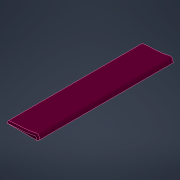
# Autodesk Inventor part: RightBackCushion
Saved by Autodesk Inventor 2021 (Build 250183000, 183)
## iProperties
Created: 2021-01-30
Part Number: RightBackCushion
Material: Generic
Document SubType Name: Modeling
Designer: argon
Density: 1 g/cm^3
Appearance: Maroon Medium
Author: argon
Autodesk Inventor part; units mm, degrees
ref_plane "YZ Plane" through (0, 0, 0) normal (1, 0, 0) x (0, 1, 0)
ref_plane "XZ Plane" through (0, 0, 0) normal (0, 1, 0) x (-1, 0, 0)
ref_plane "XY Plane" through (0, 0, 0) normal (0, 0, 1) x (1, 0, 0)
sketch "Sketch1" plane through (0, 0, 0) normal (0, 0, 1) x (1, 0, 0)
  line L0 (0, 0) -> (200, 0)
  line L1 (0, 0) -> (0, 10)
  line L2 (0, 10) -> (35.0237, 15.2953) construction
  line L3 (35.0237, 15.2953) -> (144.4747, 12.6477) construction
  line L4 (144.4747, 12.6477) -> (177.6006, 33.3111) construction
  line L5 (177.6006, 33.3111) -> (200, 33.3111) construction
  line L6 (200, 33.3111) -> (200, 0) construction
  spline S0 degree 4 poles (0, 10) (35.0237, 15.2953) (144.4747, 12.6477) (177.6006, 33.3111) (200, 33.3111) (200, 0) knots 1 1 1 1 1 2 3 3 3 3 3
  dimension "d0" = 200
  dimension "d1" = 10
  constraints: 4 end point, 2 vertical, 1 horizontal, 3 other
  measures "d0" distance of L0.start L0.end
  measures "d1" distance of L0.start L1.end
extrude "Extrusion1" add sketch "Sketch1" along normal blind 880
fillet "Fillet1" radius 10 1 edges at (150.1562, 23.3103, 880)
body "Solid1"
